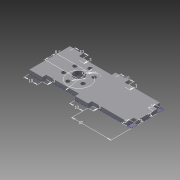
# Autodesk Inventor part: Motor mount
Saved by Autodesk Inventor 2015 (Build 190159000, 159)
## iProperties
Created: 2014-07-26
Part Number: Motor mount
Material: Generic
Document SubType Name: Modeling
Designer: karl
Density: 1 g/cm^3
Appearance: Default
Author: karl
Autodesk Inventor part; units mm, degrees
ref_plane "YZ Plane" through (0, 0, 0) normal (1, 0, 0) x (0, 1, 0)
ref_plane "XZ Plane" through (0, 0, 0) normal (0, 1, 0) x (-1, 0, 0)
ref_plane "XY Plane" through (0, 0, 0) normal (0, 0, 1) x (1, 0, 0)
sketch "Sketch1" plane through (0, 0, 0) normal (0, 0, 1) x (1, 0, 0)
  circle A0 centre (0, 0) radius 12.5 construction
  circle A1 centre (0, 8.5) radius 1.5 construction
  circle A2 centre (-7.3612, 4.25) radius 1.5 construction
  circle A3 centre (-7.3612, -4.25) radius 1.5 construction
  circle A4 centre (0, -8.5) radius 1.5 construction
  circle A5 centre (7.3612, -4.25) radius 1.5 construction
  circle A6 centre (7.3612, 4.25) radius 1.5 construction
  circle A7 centre (0, 0) radius 4 construction
  line L0 (45, -12.5) -> (-22.5, -12.5) construction
  line L1 (-22.5, -12.5) -> (-22.5, 12.5) construction
  line L2 (-22.5, 12.5) -> (45, 12.5) construction
  line L3 (45, 12.5) -> (45, -12.5) construction
  line L4 (45, -12.5) -> (-22.5, 12.5) construction
  line L5 (-22.5, -12.5) -> (45, 12.5) construction
  line L6 (-22.5, -12.5) -> (-12.5, -12.5) construction
  line L7 (-12.5, -12.5) -> (-12.5, -15.5) construction
  line L8 (-12.5, -15.5) -> (-22.5, -15.5) construction
  line L9 (-22.5, -15.5) -> (-22.5, -12.5) construction
  line L10 (12.5, -12.5) -> (22.5, -12.5) construction
  line L11 (22.5, -12.5) -> (22.5, -15.5) construction
  line L12 (22.5, -15.5) -> (12.5, -15.5) construction
  line L13 (12.5, -15.5) -> (12.5, -12.5) construction
  line L14 (-22.5, 12.5) -> (-12.5, 12.5) construction
  line L15 (-12.5, 12.5) -> (-12.5, 15.5) construction
  line L16 (-12.5, 15.5) -> (-22.5, 15.5) construction
  line L17 (-22.5, 15.5) -> (-22.5, 12.5) construction
  line L18 (12.5, 12.5) -> (22.5, 12.5) construction
  line L19 (22.5, 12.5) -> (22.5, 15.5) construction
  line L20 (22.5, 15.5) -> (12.5, 15.5) construction
  line L21 (12.5, 15.5) -> (12.5, 12.5) construction
  line L22 (45, 12.5) -> (42, 12.5) construction
  line L23 (42, 12.5) -> (42, 7.5) construction
  line L24 (42, 7.5) -> (45, 7.5) construction
  line L25 (45, 7.5) -> (45, 12.5) construction
  line L26 (45, -12.5) -> (42, -12.5) construction
  line L27 (42, -12.5) -> (42, -7.5) construction
  line L28 (42, -7.5) -> (45, -7.5) construction
  line L29 (45, -7.5) -> (45, -12.5) construction
  point P0 (11.25, 0)
  dimension "d0" = 25
  dimension "d1" = 3
  dimension "d2" = 8.5
  dimension "d5" = 360
  dimension "d7" = 8
  dimension "d8" = 10
  dimension "d9" = 3
  dimension "d10" = 10
  dimension "d11" = 3
  dimension "d12" = 22.5
  dimension "d13" = 10
  dimension "d14" = 3
  dimension "d15" = 10
  dimension "d16" = 3
  dimension "d17" = 3
  dimension "d18" = 5
  dimension "d19" = 3
  dimension "d20" = 5
  constraints: 60 end point, 14 parallel, 8 centre point, 7 horizontal, 7 perpendicular, 4 tangent, 2 coincident, 2 midpoint, 2 point on line, 1 collinear, 1 vertical alignment, 13 other
  measures "d0" diameter of A0
  measures "d1" diameter of A1
  measures "d2" distance of A1.centre point (0, 0)
  measures "d7" diameter of A7
  measures "d8" distance of L7.end L8.end
  measures "d9" distance of L6.end L7.end
  measures "d10" distance of L11.end L12.end
  measures "d11" distance of L10.end L11.end
  measures "d12" distance between parallel lines of L11 L3
  measures "d13" distance of L16.end L15.end
  measures "d14" distance of L15.end L14.end
  measures "d15" distance of L20.end L19.end
  measures "d16" distance of L19.end L18.end
  measures "d17" distance of L24.end L23.end
  measures "d18" distance of L23.end L22.end
  measures "d19" distance of L27.end L28.end
  measures "d20" distance of L26.end L27.end
sketch "Sketch2" plane through (0, 0, 0) normal (0, 0, 1) x (1, 0, 0)
  line L0 (45, -12.5) -> (-22.5, -12.5) construction
  line L1 (-22.5, -12.5) -> (-22.5, 12.5) construction
  line L2 (-22.5, 12.5) -> (45, 12.5) construction
  line L3 (-22.5, 12.5) -> (45, 12.5)
  line L4 (45, 12.5) -> (45, -12.5)
  line L5 (45, -12.5) -> (-22.5, -12.5)
  line L6 (-22.5, -12.5) -> (-22.5, 12.5)
  point P0 (0, 0)
  constraints: 8 end point, 2 parallel, 1 horizontal, 1 perpendicular
extrude "Extrusion1" add sketch "Sketch2" along normal blind 3
sketch "Sketch3" plane through (0, 0, 0) normal (0, 0, -1) x (-1, 0, 0)
  line L0 (12.5, 15.5) -> (22.5, 15.5) construction
  line L1 (12.5, 12.5) -> (12.5, 15.5) construction
  line L2 (22.5, 12.5) -> (12.5, 12.5)
  line L3 (12.5, 12.5) -> (12.5, 15.5)
  line L4 (12.5, 15.5) -> (22.5, 15.5)
  line L5 (22.5, 15.5) -> (22.5, 12.5)
  line L6 (-22.5, 15.5) -> (-12.5, 15.5) construction
  line L7 (-22.5, 12.5) -> (-22.5, 15.5) construction
  line L8 (-12.5, 15.5) -> (-12.5, 12.5) construction
  line L9 (-12.5, 12.5) -> (-22.5, 12.5)
  line L10 (-22.5, 12.5) -> (-22.5, 15.5)
  line L11 (-22.5, 15.5) -> (-12.5, 15.5)
  line L12 (-12.5, 15.5) -> (-12.5, 12.5)
  point P0 (0, 0)
  constraints: 16 end point, 4 parallel, 2 horizontal, 2 perpendicular
extrude "Extrusion2" add sketch "Sketch3" against normal blind 3
sketch "Sketch4" plane through (0, 0, 0) normal (0, 0, -1) x (-1, 0, 0)
  line L0 (-42, 12.5) -> (-42, 7.5) construction
  line L1 (-42, 7.5) -> (-45, 7.5) construction
  line L2 (-45, 12.5) -> (-42, 12.5)
  line L3 (-42, 12.5) -> (-42, 7.5)
  line L4 (-42, 7.5) -> (-45, 7.5)
  line L5 (-45, 7.5) -> (-45, 12.5)
  point P0 (0, 0)
  constraints: 8 end point, 2 parallel, 1 horizontal, 1 perpendicular
extrude "Extrusion3" cut sketch "Sketch4" against normal blind 3
sketch "Sketch5" plane through (0, 0, 0) normal (0, 0, -1) x (-1, 0, 0)
  circle A0 centre (0, 0) radius 4 construction
  circle A1 centre (0, 8.5) radius 1.5 construction
  circle A2 centre (0, 0) radius 4
  constraints: 1 centre point, 1 coincident, 1 concentric
extrude "Extrusion4" cut sketch "Sketch5" against normal blind 3
sketch "Sketch6" plane through (0, 0, 0) normal (0, 0, -1) x (-1, 0, 0)
  circle A0 centre (0, 8.5) radius 1.5 construction
  circle A1 centre (0, 8.5) radius 1.5
  point P0 (0, 0)
  constraints: 1 centre point, 1 coincident, 1 concentric
extrude "Extrusion5" cut sketch "Sketch6" against normal blind 3
mirror "Mirror1" about plane through (0, 0, 0) normal (0, 1, 0) of "Extrusion2", "Extrusion3"
pattern_circular "Circular Pattern1" count 6 over 360 about axis through (0, 0, 0) along (0, 0, 1) of "Extrusion5"
sketch "Sketch7" plane through (0, 0, 0) normal (0, 0, -1) x (-1, 0, 0)
  line L0 (12.5, 5) -> (15.5, 5)
  line L1 (15.5, 5) -> (15.5, -5)
  line L2 (15.5, -5) -> (12.5, -5)
  line L3 (12.5, -5) -> (12.5, 5)
  line L4 (12.5, 15.5) -> (12.5, 12.5) projected
  line L5 (22.5, -15.5) -> (22.5, 15.5) projected
  line L6 (-12.5, 5) -> (-15.5, 5)
  line L7 (-15.5, 5) -> (-15.5, -5)
  line L8 (-15.5, -5) -> (-12.5, -5)
  line L9 (-12.5, -5) -> (-12.5, 5)
  line L10 (-12.5, 12.5) -> (-12.5, 15.5) projected
  point P0 (0, 0)
  point P1 (15.5, 0)
  point P2 (22.5, 0)
  dimension "d34" = 3
  dimension "d35" = 10
  dimension "d36" = 3
  dimension "d37" = 10
  constraints: 16 end point, 4 parallel, 3 collinear, 2 horizontal, 2 midpoint, 2 perpendicular, 1 horizontal alignment
  measures "d34" distance of L1.end L2.end
  measures "d35" distance of L0.end L1.end
  measures "d36" distance of L8.end L7.end
  measures "d37" distance of L7.end L6.end
extrude "Extrusion6" cut sketch "Sketch7" against normal blind 3
body "Solid1"
